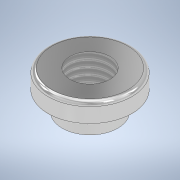
# Autodesk Inventor part: ClinchingNut_M3T1.5_Slab1.4
Saved by Autodesk Inventor 2022.2 (Build 262287000, 287)
## iProperties
Created: 2022-02-17
Part Number: ClinchingNut_M3T1.5_Slab1.4
Material: 一般
Document SubType Name: Modeling
Designer: Yuta Fujiyama
Density: 1 g/cm^3
Appearance: クローム - つや出し
Author: Yuta Fujiyama
Autodesk Inventor part; units mm, degrees
ref_plane "YZ Plane" through (0, 0, 0) normal (1, 0, 0) x (0, 1, 0)
ref_plane "XZ Plane" through (0, 0, 0) normal (0, 1, 0) x (-1, 0, 0)
ref_plane "XY Plane" through (0, 0, 0) normal (0, 0, 1) x (1, 0, 0)
sketch "スケッチ1" plane through (0, 0, 0) normal (0, 1, 0) x (-1, 0, 0)
  circle A0 centre (0, 0) radius 3.15
  dimension "d0" = 6.3
  constraints: 1 centre point, 1 coincident
  measures "d0" diameter of A0
extrude "押し出し1" add sketch "スケッチ1" along normal blind 1.5
sketch "スケッチ2" plane through (0, 0, 0) normal (0, -1, 0) x (1, 0, 0)
  circle A0 centre (0, 0) radius 2.1
  dimension "d3" = 4.2
  constraints: 1 centre point, 1 coincident
  measures "d3" diameter of A0
extrude "押し出し2" add sketch "スケッチ2" along normal blind 1.38
sketch "スケッチ3" plane through (0, 1.5, 0) normal (0, 1, 0) x (1, 0, 0)
  point P0 (0, 0)
  point P1 (0, 0)
  constraints: 1 coincident
hole "穴1" at (0, 1.5, 0) direction (0, -1, 0) diameter 3 end through all
thread "ねじ1" size "M3x0.5" class "6H" standard "ANSI Metric M Profile" full length
fillet "フィレット1" radius 0.3 1 edges at (3.15, 1.5, 0)
fillet "フィレット1" radius 0.1 1 edges at (3.15, 0, 0)
sketch "スケッチ4" plane through (0, 0, 0) normal (1, 0, 0) x (0, 1, 0)
  line L0 (-1.38, 2.1) -> (-1.38, -2.1) projected
  line L1 (-1.38, 2.1) -> (-0.58, 1.9)
  line L2 (-0.58, 1.9) -> (-0.58, 2.1)
  line L3 (-0.58, 2.1) -> (-1.38, 2.1)
  line L4 (-1.956, 0) -> (2.076, 0) projected
  point P0 (0, 0)
  dimension "d17" = 0.8
  dimension "d18" = 0.2
  constraints: 6 end point, 1 perpendicular, 1 vertical
  measures "d17" distance of L2.end L0.start
  measures "d18" distance of L1.end L2.end
revolve "回転1" cut sketch "スケッチ4" angle 360 about axis through (0, -10, 0) along (0, 1, 0)
